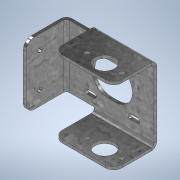
# Autodesk Inventor part: Z Drive Mount
Saved by Autodesk Inventor 2022 (Build 260153000, 153)
## iProperties
Created: 2021-10-05
Part Number: Z Drive Mount
Material: Generic
Document SubType Name: Sheet Metal
Designer: Administrator
Density: 1 g/cm^3
Appearance: Steel Galvanized
Sheet Metal Rule: 0.08in
Flat Pattern Width: 9.25003 cm
Flat Pattern Length: 10.9937 cm
Flat Pattern Area: 101.692 cm^2
Sheet Metal Width: 92.500 mm
Sheet Metal Length: 109.937 mm
Sheet Metal Area: 10169.161 mm^2
Title: Z Drive Mount v7
Author: Administrator
Autodesk Inventor part; units mm, degrees
note: some values were not read from the file. Chosen so that the rebuilt part matches the saved one: direction of "Hole2"; direction of "Hole3".
ref_plane "YZ Plane" through (0, 0, 0) normal (1, 0, 0) x (0, 1, 0)
ref_plane "XZ Plane" through (0, 0, 0) normal (0, 1, 0) x (-1, 0, 0)
ref_plane "XY Plane" through (0, 0, 0) normal (0, 0, 1) x (1, 0, 0)
sketch "Sketch1" plane through (0, 0, 0) normal (0, 0, 1) x (1, 0, 0)
  line L0 (0, 0) -> (63, 0)
  line L1 (63, 0) -> (63, 55)
  line L2 (63, 55) -> (0, 55)
  line L3 (0, 55) -> (0, 0)
  line L4 (48.5, 43) -> (48.5, 55) construction
  line L5 (48.5, 12) -> (48.5, 0) construction
  line L6 (63, 55) -> (30, 55) construction
  line L7 (30, 0) -> (63, 0) construction
  line L8 (63, 0) -> (63, 55) construction
  line L9 (15, 43) -> (20, 43) construction
  line L10 (15, 44.7) -> (20, 44.7)
  line L11 (20, 41.3) -> (15, 41.3)
  arc A0 (15, 44.7) -> (15, 41.3) centre (15, 43) ccw
  arc A1 (20, 41.3) -> (20, 44.7) centre (20, 43) ccw
  line L12 (46, 43) -> (51, 43) construction
  line L13 (46, 41.3) -> (51, 41.3)
  line L14 (51, 44.7) -> (46, 44.7)
  arc A2 (46, 44.7) -> (46, 41.3) centre (46, 43) ccw
  arc A3 (51, 41.3) -> (51, 44.7) centre (51, 43) ccw
  line L15 (15, 12) -> (20, 12) construction
  line L16 (15, 10.3) -> (20, 10.3)
  line L17 (20, 13.7) -> (15, 13.7)
  arc A4 (15, 13.7) -> (15, 10.3) centre (15, 12) ccw
  arc A5 (20, 10.3) -> (20, 13.7) centre (20, 12) ccw
  line L18 (46, 12) -> (51, 12) construction
  line L19 (46, 13.7) -> (51, 13.7)
  line L20 (51, 10.3) -> (46, 10.3)
  arc A6 (46, 13.7) -> (46, 10.3) centre (46, 12) ccw
  arc A7 (51, 10.3) -> (51, 13.7) centre (51, 12) ccw
  line L21 (30.5, 27.5) -> (35.5, 27.5) construction
  line L22 (30.5, 39.5) -> (35.5, 39.5)
  line L23 (35.5, 15.5) -> (30.5, 15.5)
  arc A8 (30.5, 39.5) -> (30.5, 15.5) centre (30.5, 27.5) ccw
  arc A9 (35.5, 15.5) -> (35.5, 39.5) centre (35.5, 27.5) ccw
  line L24 (48.5, 43) -> (17.5, 12) construction
  line L25 (0, 50) -> (20, 50)
  line L26 (20, 50) -> (20, 55)
  line L27 (0, 5) -> (20, 5)
  line L28 (20, 5) -> (20, 0)
  point P0 (17.5, 43)
  point P1 (33, 27.5)
  point P2 (33, 27.5)
  dimension "d1" = 55
  dimension "d8" = 31
  dimension "d9" = 31
  dimension "d10" = 31
  dimension "d11" = 1.7
  dimension "d12" = 5
  dimension "d13" = 12
  dimension "d14" = 5
  dimension "d15" = 15
  dimension "d53" = 63
  dimension "d83" = 43
  dimension "d84" = 5
  constraints: 68 end point, 20 point on circle, 20 tangent, 10 centre point, 9 parallel, 8 point on line, 6 equal length, 6 horizontal, 6 midpoint, 6 perpendicular, 3 coincident, 3 equal radius, 2 collinear, 1 vertical, 1 vertical alignment
  measures "d1" distance of L0.start L2.end
  measures "d8" distance of L24.end point (48.5, 12)
  measures "d9" distance of L24.start point (48.5, 12)
  measures "d10" distance of point (17.5, 43) L24.start
  measures "d11" radius of A3
  measures "d12" distance of L12.start L12.end
  measures "d13" radius of A8
  measures "d14" distance of L21.start L21.end
  measures "d15" distance from line of L3 L9.start
  measures "d53" distance between parallel lines of L1 L3
  measures "d83" distance between parallel lines of L8 L26
  measures "d84" distance of L25.end L26.end
extrude "Plate1" add sketch "Sketch1" along normal blind 2.032 contours L28 L27 L3 L25 L26 L2 L1 L0
sketch "Sketch6" plane through (20, 52.968, 0) normal (0, 1, 0) x (-1, 0, 0)
  line L0 (-43, 0) -> (0, 0)
  line L1 (0, 0) -> (0, 31)
  line L2 (0, 31) -> (-43, 31)
  line L3 (-43, 31) -> (-43, 0)
  constraints: 6 end point, 1 horizontal, 1 perpendicular, 1 vertical
edge flange "Flange2" height 31 angle 90 thickness 2.032 bend radius 2.032 thickness toward (0, 1, 0) relief tear relief width 2.032 relief depth 1.016 corner gap 2.032 corner form 0 edges at (41.5, 55, 2.032) (41.5, 0, 2.032) wall of the first edge with corners at (63, 52.968, 0) (20, 52.968, 0) (20, 52.968, 31) (63, 52.968, 31)
bend "Bend3"
corner "Corner2"
sketch "Sketch3" plane through (7, 0, 39.2981) normal (0, -1, 0) x (1, 0, 0)
  line L0 (62.3854, 0) -> (63, 0) construction
  circle A0 centre (39.5, -18.2981) radius 7
  line L1 (56, -39.2981) -> (13, -39.2981)
  line L2 (-7, -39.2981) -> (13, -39.2981) projected
  line L3 (13, -39.2981) -> (-7, -39.2981) projected
  line L4 (13, -39.2981) -> (56, -39.2981) projected
  line L5 (13, -8.2981) -> (56, -8.2981) projected
  line L6 (56, -8.2981) -> (56, -35.2341) projected
  point P0 (27, -18.2981)
  point P1 (52, -18.2981)
  dimension "d36" = 14
  dimension "d55" = 12.5
  dimension "d56" = 12.5
  dimension "d85" = 14
  dimension "d96" = 10
  dimension "d97" = 4
  constraints: 4 end point, 2 horizontal alignment, 1 centre point, 1 horizontal
  measures "d36" diameter of A0
  measures "d55" distance of A0.centre point (52, -18.298)
  measures "d56" distance of A0.centre point (27, -18.298)
  measures "d96" distance from line of L5 A0.centre
  measures "d97" distance from line of L6 point (52, -18.298)
extrude "Cut1" cut sketch "Sketch3" against normal through all
hole "Hole2" at (34, 0, 21) at (59, 0, 21) direction (0, 1, 0) diameter 3.4 depth 55 clearance for "Socket Head Cap Screw" size "M3" standard "Ansi Metric M Profile"
sketch "Sketch7" plane through (0, 5, 2.032) normal (-1, 0, 0) x (0, -1, 0)
  line L0 (-45, 0) -> (0, 0)
  line L1 (0, 0) -> (0, 28.968)
  line L2 (0, 28.968) -> (-45, 28.968)
  line L3 (-45, 28.968) -> (-45, 0)
  constraints: 6 end point, 1 horizontal, 1 perpendicular, 1 vertical
edge flange "Flange3" height 31 angle 90 thickness 2.032 bend radius 2.032 thickness toward (-1, 0, 0) relief tear relief width 2.032 relief depth 1.016 edges at (0, 27.5, 2.032) wall of the first edge with corners at (0, 50, 2.032) (0, 5, 2.032) (0, 5, 31) (0, 50, 31)
bend "Bend4"
corner "Corner3"
fillet "Corner Round2" radius 6 6 edges at (20, 53.984, 31) (63, 53.984, 31) (63, 1.016, 31) (20, 1.016, 31) (-1.016, 5, 31) (-1.016, 50, 31)
sketch "Sketch8" plane through (-2.032, 5, 4.064) normal (-1, 0, 0) x (0, 0, 1)
  line L0 (26.936, 39) -> (26.936, 6) construction
  line L1 (20.936, 0) -> (0, 0) construction
  line L2 (0, 45) -> (20.936, 45) construction
  point P0 (-4.064, -5)
  point P1 (16.936, 10)
  point P2 (16.936, 35)
  dimension "d109" = 10
  dimension "d110" = 10
  dimension "d111" = 10
  constraints: 1 vertical alignment
  measures "d109" distance from line of L0 point (16.936, 10)
  measures "d110" distance from line of L1 point (16.936, 10)
  measures "d111" distance from line of L2 point (16.936, 35)
hole "Hole3" at (-2.032, 15, 21) at (-2.032, 40, 21) direction (1, 0, 0) diameter 3.4 depth 2.032 clearance for "Socket Head Cap Screw" size "M3" standard "Ansi Metric M Profile"
equation "\"d8\" = d10"
equation "\"d9\" = d10"
equation "\"d41\" = Thickness"
equation "\"d16\" = Thickness"
equation "\"BendRadius\" = Thickness"
equation "\"BendReliefWidth\" = Thickness"
equation "\"BendReliefDepth\" = 0.5 * Thickness"
equation "\"CornerReliefSize\" = 4 * Thickness"
equation "\"MinimumRemnant\" = 2 * Thickness"
equation "\"TransitionRadius\" = BendRadius"
equation "\"JacobiRadiusSize\" = BendRadius"
equation "\"GapSize\" = Thickness"
equation "\"d7\" = d4"
equation "\"Thickness\" = 2.032"
equation "\"d4\" = 31"
body "Solid1"
body "Solid2"
